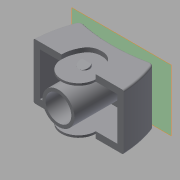
# Autodesk Inventor part: ic
Saved by Autodesk Inventor 2017 (Build 210142000, 142)
## iProperties
Created: 2017-03-16
Part Number: ic
Material: Generic
Document SubType Name: Modeling
Designer: Win10
Density: 1 g/cm^3
Appearance: Default
Author: Win10
Autodesk Inventor part; units mm, degrees
note: some values were not read from the file. Chosen so that the rebuilt part matches the saved one: direction of "Emboss1".
ref_plane "YZ Plane" through (0, 0, 0) normal (1, 0, 0) x (0, 1, 0)
ref_plane "XY Plane" through (0, 0, 0) normal (0, 0, 1) x (1, 0, 0)
sketch "Sketch1" plane through (0, 0, 0) normal (0, 1, 0) x (-1, 0, 0)
  line L0 (5.25, 3.25) -> (-5.25, 3.25)
  line L1 (-5.25, 3.25) -> (-5.25, -3.25)
  line L2 (-5.25, -3.25) -> (5.25, -3.25)
  line L3 (5.25, -3.25) -> (5.25, 3.25)
  line L4 (5.25, 3.25) -> (-5.25, -3.25) construction
  line L5 (-5.25, 3.25) -> (5.25, -3.25) construction
  point P0 (0, 0)
  dimension "d0" = 10.5
  dimension "d1" = 6.5
  constraints: 12 end point, 2 midpoint, 2 parallel, 1 horizontal, 1 perpendicular
  measures "d0" distance of L2.end L1.end
  measures "d1" distance of L1.end L0.end
extrude "Extrusion1" add sketch "Sketch1" along normal blind 4.5
sketch "Sketch2" plane through (-5.25, 0, 3.25) normal (0, 0, 1) x (1, 0, 0)
  line L0 (9.5, 4.5) -> (1, 4.5) construction
  line L1 (0, 0) -> (10.5, 0) projected
  arc A0 (1, 4.5) -> (0, 0) centre (12.9894, -0.5254) ccw
  line L2 (10.5, 0) -> (10.5, 4.5) construction
  arc A1 (10.5, 0) -> (9.5, 4.5) centre (-2.4894, -0.5254) ccw
  line L3 (-1.7976, 5.7466) -> (12.2976, 5.7466)
  line L4 (12.2976, 5.7466) -> (12.2976, -1.1573)
  line L5 (12.2976, -1.1573) -> (-1.7976, -1.1573)
  line L6 (-1.7976, -1.1573) -> (-1.7976, 5.7466)
  line L7 (-1.7976, 5.7466) -> (12.2976, -1.1573) construction
  line L8 (12.2976, 5.7466) -> (-1.7976, -1.1573) construction
  line L9 (5.25, 0) -> (5.25, 4)
  arc A2 (1, 4.5) -> (9.5, 4.5) centre (5.25, 22.3125) ccw
  point P0 (5.25, 4.5)
  point P1 (5.25, 2.2947)
  dimension "d5" = 13
  dimension "d6" = 13
  dimension "d9" = 4
  constraints: 16 end point, 7 point on circle, 4 midpoint, 3 centre point, 2 horizontal, 2 parallel, 1 perpendicular, 1 vertical, 1 vertical alignment
  measures "d5" radius of A0
  measures "d6" radius of A1
  measures "d9" distance of L9.start L9.end
extrude "Extrusion2" cut sketch "Sketch2" against normal blind 8.75
sketch "Sketch3" plane through (-5.25, 0, 3.25) normal (0, 0, 1) x (1, 0, 0)
  line L0 (5.25, 0) -> (5.25, -2) construction
  arc A0 (3.25, 0) -> (7.25, 0) centre (5.25, 0) ccw
  line L1 (5.25, 0) -> (5.25, 2.5) construction
  arc A1 (7.25, 0) -> (6.25, 2.5) centre (3.5003, -0.0499) ccw
  line L2 (10.5, 0) -> (0, 0) projected
  arc A2 (4.25, 2.5) -> (3.25, 0) centre (6.9997, -0.0499) ccw
  arc A3 (6.25, 2.5) -> (4.25, 2.5) centre (5.25, -0.3652) ccw
  dimension "d10" = 2
  dimension "d11" = 4
  dimension "d12" = 2.5
  dimension "d15" = 3.75
  dimension "d16" = 3.75
  constraints: 8 point on circle, 4 centre point, 4 end point, 2 vertical, 1 coincident, 1 point on line
  measures "d10" distance of L0.start L0.end
  measures "d11" diameter of A0
  measures "d12" distance of L1.start L1.end
  measures "d15" radius of A1
  measures "d16" radius of A2
extrude "Extrusion3" cut sketch "Sketch3" against normal blind 0.5
sketch "Sketch4" plane through (-5.25, 0, 2.75) normal (0, 0, 1) x (1, 0, 0)
  circle A0 centre (5.25, 0.65) radius 0.625
  point P0 (5.25, 0)
  dimension "d19" = 1.25
  dimension "d20" = 0.65
  constraints: 1 centre point
  measures "d19" diameter of A0
  measures "d20" distance of point (5.25, 0) A0.centre
extrude "Extrusion4" add sketch "Sketch4" along normal blind 0.35
sketch "Sketch5" plane through (0, 0, 0) normal (1, 0, 0) x (0, 1, 0)
  line L0 (1.275, 2.75) -> (1.275, 3.1) projected
  line L1 (1.275, 3.225) -> (0.0241, 2.75)
  line L2 (0, 2.75) -> (2.5, 2.75) projected
  line L3 (0.0241, 2.75) -> (-0.2515, 2.75)
  line L4 (-0.2515, 2.75) -> (-0.2515, 3.426)
  line L5 (-0.2515, 3.426) -> (1.275, 3.426)
  line L6 (1.275, 3.426) -> (1.275, 3.225)
  point P0 (0, 0)
  constraints: 10 end point, 3 perpendicular, 2 point on line, 1 horizontal
extrude "Extrusion5" cut sketch "Sketch5" along normal mid plane 1.6
fillet "Fillet1" radius 1.5 2 edges at (-1, 2.5, 3) (1, 2.5, 3)
mirror "Mirror1" about plane through (0, 0, 0) normal (0, 0, 1) of "Extrusion3", "Extrusion4", "Extrusion5", "Fillet1"
sketch "Sketch6" plane through (-5.25, 0, 2.75) normal (0, 0, 1) x (1, 0, 0)
  arc A0 (3.25, 0) -> (7.25, 0) centre (5.25, 0) ccw
  line L0 (7.25, 0) -> (3.25, 0)
  line L1 (7.25, 0) -> (3.25, 0)
  point P0 (5.25, 0)
  dimension "d26" = 4
  constraints: 4 end point, 2 point on circle, 1 centre point, 1 coincident, 1 collinear
  measures "d26" diameter of A0
extrude "Extrusion6" add sketch "Sketch6" against normal up to surface (5.5 mm away)
sketch "Sketch7" plane through (0, 0, 0) normal (0, -1, 0) x (1, 0, 0)
  line L0 (5.25, 3.25) -> (5.25, -3.25) construction
  line L1 (-5.25, -3.25) -> (-5.25, 3.25) construction
  line L2 (-5.25, -3.25) -> (5.25, -3.25) construction
  line L3 (-5.25, 3.25) -> (5.25, 3.25) construction
  line L4 (4.5, -2.5) -> (4.5, 2.5)
  line L5 (4.5, 2.5) -> (-4.5, 2.5)
  line L6 (-4.5, 2.5) -> (-4.5, -2.5)
  line L7 (-4.5, -2.5) -> (4.5, -2.5)
  point P0 (0, 0)
  dimension "d29" = 0.75
  constraints: 12 end point, 4 perpendicular, 3 other
  measures "d29" distance between parallel lines of L0 L4
extrude "Extrusion7" cut sketch "Sketch7" against normal blind 3.65 and the other way blind 2.575
sketch "Sketch8" plane through (0, 3.65, 0) normal (0, -1, 0) x (1, 0, 0)
  circle A0 centre (0, 0) radius 1.875
  dimension "d34" = 3.75
  constraints: 1 centre point, 1 coincident
  measures "d34" diameter of A0
extrude "Extrusion8" add sketch "Sketch8" along normal blind 6.5
shell "Shell1" thickness 0.375 removed faces 1 at (0.714, -2.85, -0.5844)
chamfer "Chamfer1" distance 0.6425 angle 80 2 edges at (-4.5, 3.65, 0) (4.5, 3.65, 0) measured on face at (3.625, 3.65, 0)
fillet "Fillet2" radius 0.5 2 edges at (4.25, 4.5, 0) (-4.25, 4.5, 0)
fillet "Fillet2" radius 0.2 6 edges at (0, 4, -3.25) (0, 4, 3.25) (-4.9511, 2.2947, 3.25) (-4.9511, 2.2947, -3.25) (4.9511, 2.2947, -3.25) (4.9511, 2.2947, 3.25)
ref_plane "Work Plane1" through (0, 5, 0) normal (0, 1, 0) x (-1, 0, 0)
sketch "Sketch9" plane through (0, 5, 0) normal (0, 1, 0) x (-1, 0, 0)
  line L0 (-3.2656, -1.6478) -> (-3.2656, 1.7586) construction
  line L1 (-3.2656, 1.7586) -> (0.3819, 1.7586) construction
  line L2 (0.3819, 1.7586) -> (0.3819, -1.6478) construction
  line L3 (0.3819, -1.6478) -> (-3.2656, -1.6478) construction
  line L4 (-0.7656, 0.5386) -> (-0.7656, -0.4298)
  line L5 (-0.7656, -0.4298) -> (-1.0209, -0.4298)
  line L6 (-1.0209, -0.4298) -> (-1.0209, -0.1117)
  line L7 (-1.0209, -0.1117) -> (-3.0104, -0.1117)
  line L8 (-3.0104, -0.1117) -> (-3.0104, -0.4298)
  line L9 (-3.0104, -0.4298) -> (-3.2656, -0.4298)
  line L10 (-3.2656, -0.4298) -> (-3.2656, 0.5386)
  line L11 (-3.2656, 0.5386) -> (-3.0104, 0.5386)
  line L12 (-3.0104, 0.5386) -> (-3.0104, 0.2205)
  line L13 (-3.0104, 0.2205) -> (-1.0209, 0.2205)
  line L14 (-1.0209, 0.2205) -> (-1.0209, 0.5386)
  line L15 (-1.0209, 0.5386) -> (-0.7656, 0.5386)
  spline S0 degree 2 poles (1.1362, 0.8607) (1.3023, 1.0026) (1.7886, 1.1606) (2.1006, 1.1606) knots 0 0 0 1 2 2 2
  spline S1 degree 2 poles (2.1006, 1.1606) (2.4044, 1.1606) (2.8967, 1.0066) (3.0629, 0.8607) knots 0 0 0 1 2 2 2
  spline S2 degree 2 poles (3.0629, 0.8607) (3.2371, 0.7068) (3.4032, 0.2996) (3.4032, 0.0544) knots 0 0 0 1 2 2 2
  spline S3 degree 2 poles (3.4032, 0.0544) (3.4032, -0.1988) (3.231, -0.604) (3.0629, -0.7519) knots 0 0 0 1 2 2 2
  spline S4 degree 2 poles (3.0629, -0.7519) (2.8967, -0.8957) (2.4085, -1.0497) (2.1006, -1.0497) knots 0 0 0 1 2 2 2
  spline S5 degree 2 poles (2.1006, -1.0497) (1.7865, -1.0497) (1.3084, -0.8937) (1.1362, -0.7499) knots 0 0 0 1 2 2 2
  spline S6 degree 2 poles (1.1362, -0.7499) (0.9701, -0.604) (0.7979, -0.1968) (0.7979, 0.0544) knots 0 0 0 1 2 2 2
  spline S7 degree 2 poles (0.7979, 0.0544) (0.7979, 0.3097) (0.9762, 0.7189) (1.1362, 0.8607) knots 0 0 0 1 2 2 2
  spline S8 degree 2 poles (2.1006, 0.8141) (1.8534, 0.8141) (1.4705, 0.7068) (1.3449, 0.6095) knots 0 0 0 1 2 2 2
  spline S9 degree 2 poles (1.3449, 0.6095) (1.2152, 0.5103) (1.0856, 0.2307) (1.0856, 0.0564) knots 0 0 0 1 2 2 2
  spline S10 degree 2 poles (1.0856, 0.0564) (1.0856, -0.1239) (1.2112, -0.3953) (1.3449, -0.4987) knots 0 0 0 1 2 2 2
  spline S11 degree 2 poles (1.3449, -0.4987) (1.4725, -0.5979) (1.8574, -0.7033) (2.1006, -0.7033) knots 0 0 0 1 2 2 2
  spline S12 degree 2 poles (2.1006, -0.7033) (2.5929, -0.7033) (3.1155, -0.29) (3.1155, 0.0564) knots 0 0 0 1 2 2 2
  spline S13 degree 2 poles (3.1155, 0.0564) (3.1155, 0.4029) (2.5929, 0.8141) (2.1006, 0.8141) knots 0 0 0 1 2 2 2
  point P0 (0, 0)
  constraints: 2 other
emboss "Emboss1" sketch "Sketch9" operation add depth 0.1 direction (0, -1, 0)
body "Solid1"
